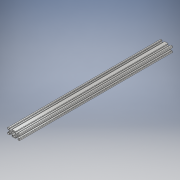
# Autodesk Inventor part: Aluminium Profile 2040 500mm
Saved by Autodesk Inventor 2019 (Build 230136000, 136)
## iProperties
Created: 2020-11-22
Part Number: Aluminium Profile 2040 500mm
Material: Aluminum 6061
Document SubType Name: Modeling
Designer: asus
Density: 2.7 g/cm^3
Appearance: Aluminum - Polished
Author: asus
Autodesk Inventor part; units mm, degrees
ref_plane "YZ Plane" through (0, 0, 0) normal (1, 0, 0) x (0, 1, 0)
ref_plane "XZ Plane" through (0, 0, 0) normal (0, 1, 0) x (-1, 0, 0)
ref_plane "XY Plane" through (0, 0, 0) normal (0, 0, 1) x (1, 0, 0)
sketch "Sketch1" plane through (0, 0, 0) normal (0, 0, 1) x (1, 0, 0)
  line L0 (-33.69, 10) -> (-33.9, 10.21)
  line L1 (-33.9, 10.21) -> (-33.9, 12.8393)
  line L2 (-33.9, 12.8393) -> (-36.5607, 15.5)
  line L3 (-36.5607, 15.5) -> (-38.2, 15.5)
  line L4 (-38.2, 15.5) -> (-38.2, 13.395)
  line L5 (-38.2, 13.395) -> (-38.815, 13.395)
  line L6 (-38.815, 13.395) -> (-40, 14.58)
  line L7 (-40, 14.58) -> (-40, 18.5)
  arc A0 (-38.5, 20) -> (-40, 18.5) centre (-38.5, 18.5) ccw
  line L8 (-38.5, 20) -> (-34.58, 20)
  line L9 (-34.58, 20) -> (-33.395, 18.815)
  line L10 (-33.395, 18.815) -> (-33.395, 18.2)
  line L11 (-33.395, 18.2) -> (-35.5, 18.2)
  line L12 (-35.5, 18.2) -> (-35.5, 16.5607)
  line L13 (-35.5, 16.5607) -> (-32.8393, 13.9)
  line L14 (-32.8393, 13.9) -> (-30.21, 13.9)
  line L15 (-30.21, 13.9) -> (-30, 13.69)
  line L16 (-30, 13.69) -> (-29.79, 13.9)
  line L17 (-29.79, 13.9) -> (-27.1607, 13.9)
  line L18 (-27.1607, 13.9) -> (-24.5, 16.5607)
  line L19 (-24.5, 16.5607) -> (-24.5, 18.2)
  line L20 (-24.5, 18.2) -> (-26.605, 18.2)
  line L21 (-26.605, 18.2) -> (-26.605, 18.815)
  line L22 (-26.605, 18.815) -> (-25.42, 20)
  line L23 (-25.42, 20) -> (-20, 20)
  line L24 (-20, 18.2) -> (-22.7, 18.2)
  line L25 (-22.7, 18.2) -> (-22.7, 16.2393)
  line L26 (-22.7, 16.2393) -> (-26.1, 12.8393)
  line L27 (-26.1, 12.8393) -> (-26.1, 10)
  circle A1 centre (-30, 10) radius 2.3
  line L28 (-24.5, 1.8) -> (-26.605, 1.8)
  line L29 (-24.5, 3.4393) -> (-24.5, 1.8)
  line L30 (-22.7, 3.7607) -> (-26.1, 7.1607)
  line L31 (-22.7, 1.8) -> (-22.7, 3.7607)
  line L32 (-29.79, 6.1) -> (-27.1607, 6.1)
  line L33 (-30, 6.31) -> (-29.79, 6.1)
  line L34 (-30.21, 6.1) -> (-30, 6.31)
  line L35 (-32.8393, 6.1) -> (-30.21, 6.1)
  line L36 (-33.9, 9.79) -> (-33.9, 7.1607)
  line L37 (-33.69, 10) -> (-33.9, 9.79)
  line L38 (-26.1, 7.1607) -> (-26.1, 10)
  line L39 (-27.1607, 6.1) -> (-24.5, 3.4393)
  line L40 (-33.395, 1.185) -> (-33.395, 1.8)
  line L41 (-35.5, 3.4393) -> (-32.8393, 6.1)
  line L42 (-33.395, 1.8) -> (-35.5, 1.8)
  line L43 (-35.5, 1.8) -> (-35.5, 3.4393)
  line L44 (-34.58, 0) -> (-33.395, 1.185)
  line L45 (-33.9, 7.1607) -> (-36.5607, 4.5)
  line L46 (-36.5607, 4.5) -> (-38.2, 4.5)
  line L47 (-38.2, 4.5) -> (-38.2, 6.605)
  line L48 (-38.2, 6.605) -> (-38.815, 6.605)
  line L49 (-38.815, 6.605) -> (-40, 5.42)
  line L50 (-38.5, 0) -> (-34.58, 0)
  arc A2 (-40, 1.5) -> (-38.5, 0) centre (-38.5, 1.5) ccw
  line L51 (-40, 5.42) -> (-40, 1.5)
  line L52 (-26.605, 1.8) -> (-26.605, 1.185)
  line L53 (-20, 1.8) -> (-22.7, 1.8)
  line L54 (-25.42, 0) -> (-20, 0)
  line L55 (-26.605, 1.185) -> (-25.42, 0)
  line L56 (-15.5, 18.2) -> (-13.395, 18.2)
  line L57 (-15.5, 16.5607) -> (-15.5, 18.2)
  line L58 (-17.3, 16.2393) -> (-13.9, 12.8393)
  line L59 (-17.3, 18.2) -> (-17.3, 16.2393)
  line L60 (-10.21, 13.9) -> (-12.8393, 13.9)
  line L61 (-10, 13.69) -> (-10.21, 13.9)
  line L62 (-9.79, 13.9) -> (-10, 13.69)
  line L63 (-7.1607, 13.9) -> (-9.79, 13.9)
  line L64 (-6.1, 10.21) -> (-6.1, 12.8393)
  line L65 (-6.31, 10) -> (-6.1, 10.21)
  line L66 (-13.9, 12.8393) -> (-13.9, 10)
  circle A3 centre (-10, 10) radius 2.3
  line L67 (-12.8393, 13.9) -> (-15.5, 16.5607)
  line L68 (-6.605, 18.815) -> (-6.605, 18.2)
  line L69 (-4.5, 16.5607) -> (-7.1607, 13.9)
  line L70 (-6.605, 18.2) -> (-4.5, 18.2)
  line L71 (-4.5, 18.2) -> (-4.5, 16.5607)
  line L72 (-5.42, 20) -> (-6.605, 18.815)
  line L73 (-6.1, 12.8393) -> (-3.4393, 15.5)
  line L74 (-3.4393, 15.5) -> (-1.8, 15.5)
  line L75 (-1.8, 15.5) -> (-1.8, 13.395)
  line L76 (-1.8, 13.395) -> (-1.185, 13.395)
  line L77 (-1.185, 13.395) -> (0, 14.58)
  line L78 (-1.5, 20) -> (-5.42, 20)
  arc A4 (0, 18.5) -> (-1.5, 20) centre (-1.5, 18.5) ccw
  line L79 (0, 14.58) -> (0, 18.5)
  line L80 (-13.395, 18.2) -> (-13.395, 18.815)
  line L81 (-20, 18.2) -> (-17.3, 18.2)
  line L82 (-14.58, 20) -> (-20, 20)
  line L83 (-13.395, 18.815) -> (-14.58, 20)
  line L84 (-15.5, 1.8) -> (-13.395, 1.8)
  line L85 (-15.5, 3.4393) -> (-15.5, 1.8)
  line L86 (-17.3, 3.7607) -> (-13.9, 7.1607)
  line L87 (-17.3, 1.8) -> (-17.3, 3.7607)
  line L88 (-20, 1.8) -> (-17.3, 1.8)
  line L89 (-14.58, 0) -> (-20, 0)
  line L90 (-13.9, 7.1607) -> (-13.9, 10)
  line L91 (-10.21, 6.1) -> (-12.8393, 6.1)
  line L92 (-10, 6.31) -> (-10.21, 6.1)
  line L93 (-9.79, 6.1) -> (-10, 6.31)
  line L94 (-12.8393, 6.1) -> (-15.5, 3.4393)
  line L95 (-6.605, 1.185) -> (-6.605, 1.8)
  line L96 (-7.1607, 6.1) -> (-9.79, 6.1)
  line L97 (-6.1, 9.79) -> (-6.1, 7.1607)
  line L98 (-6.31, 10) -> (-6.1, 9.79)
  line L99 (-4.5, 3.4393) -> (-7.1607, 6.1)
  line L100 (-6.605, 1.8) -> (-4.5, 1.8)
  line L101 (-4.5, 1.8) -> (-4.5, 3.4393)
  line L102 (-5.42, 0) -> (-6.605, 1.185)
  line L103 (-13.395, 1.8) -> (-13.395, 1.185)
  line L104 (-6.1, 7.1607) -> (-3.4393, 4.5)
  line L105 (-3.4393, 4.5) -> (-1.8, 4.5)
  line L106 (-1.8, 4.5) -> (-1.8, 6.605)
  line L107 (-1.8, 6.605) -> (-1.185, 6.605)
  line L108 (-1.5, 0) -> (-5.42, 0)
  line L109 (-1.185, 6.605) -> (0, 5.42)
  line L110 (0, 5.42) -> (0, 1.5)
  arc A5 (-1.5, 0) -> (0, 1.5) centre (-1.5, 1.5) ccw
  line L111 (-13.395, 1.185) -> (-14.58, 0)
  constraints: 224 end point, 8 point on circle, 6 centre point
extrude "Extrusion5" add sketch "Sketch1" along normal blind 500
body "Solid5"
